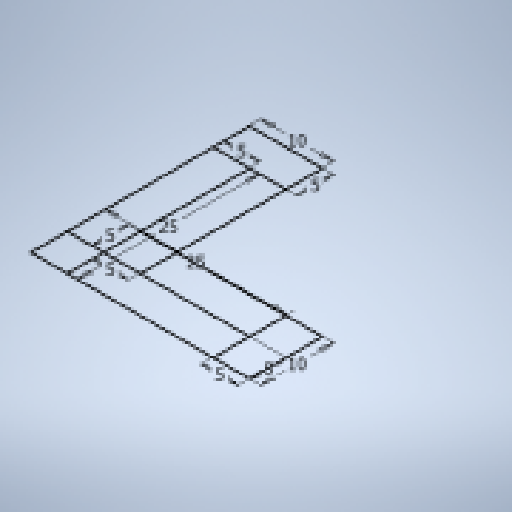
# Autodesk Inventor part: roof-joint
Saved by Autodesk Inventor 2023 (Build 270158000, 158)
## iProperties
Created: 2022-10-04
Part Number: roof-joint
Material: Generic
Document SubType Name: Modeling
Designer: carso
Density: 1 g/cm^3
Appearance: Default
Author: carso
Autodesk Inventor part; units mm, degrees
ref_plane "YZ Plane" through (0, 0, 0) normal (1, 0, 0) x (0, 1, 0)
ref_plane "XZ Plane" through (0, 0, 0) normal (0, 1, 0) x (-1, 0, 0)
ref_plane "XY Plane" through (0, 0, 0) normal (0, 0, 1) x (1, 0, 0)
sketch "Sketch1" plane through (0, 0, 0) normal (0, 1, 0) x (-1, 0, 0)
  line L0 (0, 0) -> (-25, 0)
  line L1 (-25, 0) -> (-25, -5)
  line L2 (-25, -5) -> (0, -5)
  line L3 (0, -5) -> (0, 0)
  line L4 (0, 0) -> (-5, 0)
  line L5 (-5, 0) -> (-5, -25)
  line L6 (-5, -25) -> (0, -25)
  line L7 (0, -25) -> (0, 0)
  line L8 (-25, -5) -> (-5, -5)
  line L9 (-5, -5) -> (-5, -10)
  line L10 (-5, -10) -> (-25, -10)
  line L11 (-25, -10) -> (-25, -5)
  line L12 (-5, -25) -> (-10, -25)
  line L13 (-10, -25) -> (-10, -5)
  line L14 (-10, -5) -> (-5, -5)
  line L15 (-5, -5) -> (-5, -25)
  line L16 (0, -25) -> (-10, -25)
  line L17 (-10, -25) -> (-10, -30)
  line L18 (-10, -30) -> (0, -30)
  line L19 (0, -30) -> (0, -25)
  line L20 (-25, -10) -> (-30, -10)
  line L21 (-30, -10) -> (-30, 0)
  line L22 (-30, 0) -> (-25, 0)
  line L23 (-25, 0) -> (-25, -10)
  point P0 (-10, -10)
  dimension "d0" = 25
  dimension "d1" = 5
  dimension "d2" = 5
  dimension "d3" = 25
  dimension "d4" = 5
  dimension "d5" = 5
  dimension "d6" = 10
  dimension "d7" = 5
  dimension "d8" = 5
  dimension "d9" = 10
  constraints: 48 end point, 12 parallel, 6 horizontal, 6 perpendicular, 2 point on line
  measures "d0" distance of L2.end L1.end
  measures "d1" distance of L1.end L0.end
  measures "d2" distance of L6.end L5.end
  measures "d3" distance of L5.end L4.end
  measures "d4" distance of L8.end L9.end
  measures "d5" distance of L13.end L14.end
  measures "d6" distance of L18.end L17.end
  measures "d7" distance of L17.end L16.end
  measures "d8" distance of L21.end L22.end
  measures "d9" distance of L20.end L21.end
extrude "Extrusion1" add sketch "Sketch1" along normal blind 25 contours L1 L11 L20 L21 L22 | L5 L10 L13 L2 | L19 L18 L17 L12 L6 | L2 L13 L10 L11 | L5 L12 L13 L10
body "Solid1"
